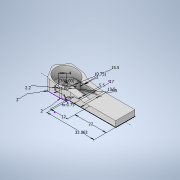
# Autodesk Inventor part: motor_arm
Saved by Autodesk Inventor 2022 (Build 260153000, 153)
## iProperties
Created: 2022-01-21
Part Number: motor_arm
Material: Generic
Document SubType Name: Modeling
Designer: felix
Density: 1 g/cm^3
Appearance: Default
Author: felix
Autodesk Inventor part; units mm, degrees
ref_plane "YZ Plane" through (0, 0, 0) normal (1, 0, 0) x (0, 1, 0)
ref_plane "XZ Plane" through (0, 0, 0) normal (0, 1, 0) x (-1, 0, 0)
ref_plane "XY Plane" through (0, 0, 0) normal (0, 0, 1) x (1, 0, 0)
sketch "Sketch1" plane through (0, 0, 0) normal (0, 1, 0) x (-1, 0, 0)
  line L0 (-0.9057, -9.2473) -> (-7.4436, -5.5611)
  line L1 (-8.4613, -3.8393) -> (-8.5382, 3.7052)
  line L2 (8.4608, 3.8848) -> (8.5378, -3.6659)
  line L3 (7.5556, -5.408) -> (1.0942, -9.2269)
  circle A0 centre (0, 0) radius 7.75
  circle A1 centre (0, 0) radius 2.75
  line L4 (0, 0) -> (2.8284, -2.8284)
  line L5 (0, 0) -> (4, 0) construction
  circle A2 centre (2.8284, -2.8284) radius 1.1
  circle A3 centre (0, 0) radius 1
  circle A4 centre (2.8284, 2.8284) radius 1.1
  circle A5 centre (-2.8284, 2.8284) radius 1.1
  circle A6 centre (-2.8284, -2.8284) radius 1.1
  line L6 (0, -18) -> (0, 46) construction
  line L7 (6.75, 9.4666) -> (6.75, 41.2457)
  line L8 (-6.75, 9.4666) -> (-6.75, 41.2457)
  arc A7 (7.5556, -5.408) -> (8.5378, -3.6659) centre (6.538, -3.6863) ccw
  arc A8 (-0.9057, -9.2473) -> (1.0942, -9.2269) centre (0.0766, -7.5052) ccw
  arc A9 (-8.4613, -3.8393) -> (-7.4436, -5.5611) centre (-6.4614, -3.8189) ccw
  arc A10 (6.75, 9.4666) -> (8.2128, 4.8292) centre (19.046, 10.7958) ccw
  arc A11 (8.4608, 3.8848) -> (8.2128, 4.8292) centre (6.4609, 3.8644) ccw
  arc A12 (-8.2794, 4.7097) -> (-6.75, 9.4666) centre (-19.046, 10.7958) ccw
  arc A13 (-8.2794, 4.7097) -> (-8.5382, 3.7052) centre (-6.5384, 3.7256) ccw
  line L9 (2.75, 7.2457) -> (2.75, 8.1823)
  line L10 (-2.75, 7.2457) -> (-2.75, 8.1823)
  line L11 (2.75, 8.1823) -> (2.75, 19.2457)
  line L12 (-2.75, 8.1823) -> (-2.75, 19.2457)
  line L13 (-0.0003, 9.815) -> (0, 9.8148)
  line L14 (2.75, 8.2755) -> (8.0834, 5.0337)
  line L15 (-6.75, 41.2457) -> (6.75, 41.2457)
  line L16 (-2.75, 19.2457) -> (2.75, 19.2457)
  line L17 (-2.75, 19.2457) -> (-6.75, 19.2457)
  line L18 (2.75, 19.2457) -> (6.75, 19.2457)
  line L19 (2.75, 19.2457) -> (2.75, 41.2457)
  line L20 (-2.75, 19.2457) -> (-2.75, 41.2457)
  line L21 (-2.75, 8.2755) -> (-8.0834, 5.0337)
  line L22 (8.0834, 5.0337) -> (8.1117, 5.0165)
  line L23 (-8.0834, 5.0337) -> (-8.1117, 5.0165)
  point P0 (0.1001, -9.8144)
  point P1 (-8.4495, -4.9939)
  point P2 (8.5496, -4.8205)
  point P3 (-2.75, 8.2483)
  point P4 (-2.75, 7.2457)
  dimension "d1" = 15.5
  dimension "d0" = 17
  dimension "d2" = 0.75
  dimension "d3" = 5.5
  dimension "d4" = 4
  dimension "d5" = 45
  dimension "d6" = 2.2
  dimension "d7" = 2
  dimension "d10" = 360
  dimension "d13" = 2
  dimension "d14" = 2
  dimension "d15" = 2
  dimension "d16" = 13.5
  dimension "d17" = 5.5
  dimension "d19" = 12
  dimension "d61" = 22
  dimension "d62" = 33.0633
  dimension "d63" = 0.75
  constraints: 48 end point, 16 point on circle, 14 point on line, 13 centre point, 10 symmetric about line, 10 tangent, 7 coincident, 4 perpendicular, 4 vertical, 2 equal radius, 2 horizontal, 1 equal length, 21 other
  measures "d0" distance between parallel lines of L1 L2
  measures "d3" diameter of A1
  measures "d4" distance of L4.start L4.end
  measures "d5" angle of L4 L5
  measures "d6" diameter of A2
  measures "d7" diameter of A3
  measures "d13" radius of A7
  measures "d14" radius of A11
  measures "d15" radius of A13
  measures "d16" distance between parallel lines of L8 L7
  measures "d17" distance between parallel lines of L10 L9
  measures "d19" distance of L11.end L9.start
  measures "d61" distance of L11.end L19.end
  measures "d62" distance of L19.end L9.end
extrude "Extrusion1_arm1" add sketch "Sketch1" along normal blind 1 contours L12 L16 L11 L9 A0 L10
extrude "Extrusion2_arm1" add sketch "Sketch1" along normal blind 4 contours L8 L15 L20 L17 | L18 L19 L15 L7
extrude "Extrusion3_arm1" add sketch "Sketch1" along normal blind 4 contours L20 L15 L19 L16
extrude "Extrusion4_arm1" cut sketch "Sketch1" along normal blind 4 contours L12 L16 L11 L9 A0 L10
ref_plane "Work Plane2_arm1" through (6.75, 4, 19.2457) normal (0, 0.9862856, 0.1650476) x (-1, 0, 0)
extrude "Extrusion15_arm1" cut sketch "Sketch1" along normal blind 8 contours L0 A9 L1 A13 A12 L23 L21 L12 L10 A0 L9 L11 L14 L22 A10 A11 L2 A7 L3 A8 | A12 L8 L17 L12 L21 L23 | L22 L14 L11 L18 L7 A10 | L8 L15 L20 L17 | L12 L16 L11 L9 A0 L10 | L20 L15 L19 L16 | L18 L19 L15 L7 | A0 | A1 | A2 | A3 | A4 | A5 | A6
extrude "Extrusion16_arm1" add sketch "Sketch1" along normal up to surface contours L0 A9 L1 A13 A12 L23 L21 L12 L10 A0 L9 L11 L14 L22 A10 A11 L2 A7 L3 A8 | A12 L8 L17 L12 L21 L23 | L22 L14 L11 L18 L7 A10 surface through (6.75, 4, 19.2457) normal (0, 0.9862856, 0.1650476)
ref_plane "Work Plane3_arm1" through (2.749, 4, 19.2453) normal (0, 0.9711343, -0.2385335) x (-1, 0, 0)
extrude "Extrusion17_arm1" cut sketch "Sketch1" along normal blind 10 contours L12 L16 L11 L9 A0 L10
extrude "Extrusion18_arm1" add sketch "Sketch1" against normal up to surface contours L12 L16 L11 L9 A0 L10 surface through (2.749, 4, 19.2453) normal (0, 0.9711343, -0.2385335)
extrude "Extrusion19" add sketch "Sketch1" along normal blind 1 contours A0
extrude "Extrusion20" add sketch "Sketch1" along normal blind 0.4 contours A1
extrude "Extrusion21" add sketch "Sketch1" along normal blind 4 contours L8 L15 L20 L17 | L20 L15 L19 L16 | L18 L19 L15 L7
equation "\"d63\" = d2"
body "Solid1"
